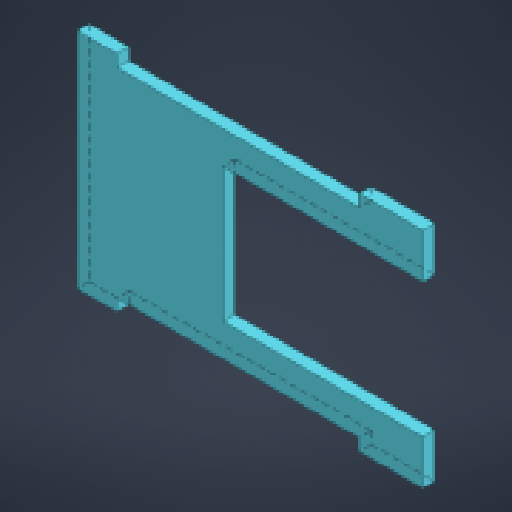
# Autodesk Inventor part: femur_reinforcement_tibea_steel
Saved by Autodesk Inventor 2026 (Build 300175000, 175)
## iProperties
Created: 2026-05-03
Part Number: femur_reinforcement_tibea_steel
Material: Сталь
Document SubType Name: Modeling
Designer: user
Density: 7.85 g/cm^3
Appearance: Серо-синий
Author: user
Autodesk Inventor part; units mm, degrees
ref_plane "YZ Plane" through (0, 0, 0) normal (1, 0, 0) x (0, 1, 0)
ref_plane "XZ Plane" through (0, 0, 0) normal (0, 1, 0) x (-1, 0, 0)
ref_plane "XY Plane" through (0, 0, 0) normal (0, 0, 1) x (1, 0, 0)
sketch "Эскиз3" plane through (0, 0, 0) normal (0, 0, 1) x (1, 0, 0)
  line L0 (15, 0) -> (106.2, 0)
  line L1 (106.2, 49.8) -> (15, 49.8)
  line L2 (0, 49.8) -> (0, 0)
  line L3 (0, 0) -> (0, -3)
  line L4 (0, -3) -> (15, -3)
  line L5 (15, -3) -> (15, 0)
  line L6 (0, 49.8) -> (0, 52.8)
  line L7 (0, 52.8) -> (15, 52.8)
  line L8 (15, 52.8) -> (15, 49.8)
  line L9 (106.2, 0) -> (106.2, -3)
  line L10 (106.2, -3) -> (110.7, -3)
  line L11 (110.7, -3) -> (110.7, 3)
  line L12 (105.7, 8) -> (47, 8)
  line L13 (42, 13) -> (42, 36.8)
  line L14 (47, 41.8) -> (105.7, 41.8)
  line L15 (110.7, 46.8) -> (110.7, 52.8)
  line L16 (110.7, 52.8) -> (106.2, 52.8)
  line L17 (106.2, 52.8) -> (106.2, 49.8)
  arc A0 (105.7, 41.8) -> (110.7, 46.8) centre (105.7, 46.8) ccw
  arc A1 (110.7, 3) -> (105.7, 8) centre (105.7, 3) ccw
  arc A2 (42, 13) -> (47, 8) centre (47, 13) ccw
  arc A3 (47, 41.8) -> (42, 36.8) centre (47, 36.8) ccw
  point P0 (110.7, 8)
  point P1 (42, 8)
  point P2 (42, 41.8)
  point P3 (110.7, 41.8)
  dimension "d8" = 49.8
  dimension "d9" = 3
  dimension "d10" = 15
  dimension "d11" = 91.2
  dimension "d12" = 42
  dimension "d13" = 4.5
  dimension "d14" = 5
  dimension "d15" = 8
  dimension "d16" = 5
  constraints: 36 end point, 13 point on line, 11 perpendicular, 8 point on circle, 8 tangent, 4 centre point, 3 equal length, 2 equal radius, 2 vertical, 1 horizontal, 1 horizontal alignment, 1 parallel, 1 vertical alignment
  measures "d8" distance between parallel lines of L1 L0
  measures "d9" distance between parallel lines of L4 L0
  measures "d10" distance between parallel lines of L3 L5
  measures "d11" distance between parallel lines of L5 L9
  measures "d12" distance between parallel lines of L2 L13
  measures "d13" distance between parallel lines of L15 L17
  measures "d14" radius of A0
  measures "d15" distance between parallel lines of L14 L1
  measures "d16" radius of A2
extrude "Выдавливание3" add sketch "Эскиз3" along normal blind 3
equation "\"d8\" = width_profile_femur - 2 * tolerance_plazma"
equation "\"d9\" = thickness_steel"
equation "\"d6\" = thickness_steel"
equation "\"tolerance_plazma\" = 0.1"
equation "\"thickness_steel\" = 3"
equation "\"d_main_screw_holes\" = 6.1"
equation "\"d_main_shaft\" = 15"
equation "\"thickness_profile_tibea\" = 3"
equation "\"hight_shaft_shift\" = 37"
equation "\"thickness_profile_femur\" = 3"
equation "\"width_shaft_shift\" = 35"
equation "\"width_flattened_surface\" = 12"
equation "\"width_profile_femur\" = 50"
